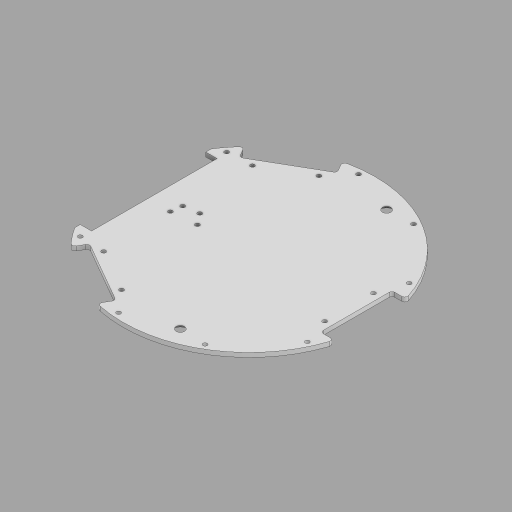
# Autodesk Inventor part: V_1
Saved by Autodesk Inventor 2024.2 (Build 282272000, 272)
## iProperties
Created: 2023-12-06
Part Number: V_1
Material: Типовые
Document SubType Name: Modeling
Designer: Фёдор
Density: 1 g/cm^3
Appearance: По умолчанию
Author: Фёдор
Autodesk Inventor part; units mm, degrees
ref_plane "YZ Plane" through (0, 0, 0) normal (1, 0, 0) x (0, 1, 0)
ref_plane "XZ Plane" through (0, 0, 0) normal (0, 1, 0) x (-1, 0, 0)
ref_plane "XY Plane" through (0, 0, 0) normal (0, 0, 1) x (1, 0, 0)
sketch "Эскиз1" plane through (0, 0, 0) normal (0, 1, 0) x (-1, 0, 0)
  arc A0 (75.6241, 45) -> (63.8377, 60.5702) centre (0, 0) ccw
  line L0 (0, 0) -> (-88, 0) construction
  line L1 (0, 0) -> (44, 76.2102) construction
  line L2 (0, 0) -> (44, -76.2102) construction
  line L3 (75.6241, 45) -> (75.6241, -45)
  arc A1 (75.6241, -45) -> (75.6241, 45) centre (0, 0) ccw construction
  line L4 (15.7099, 77.2104) -> (59.0112, 52.2104)
  line L5 (15.7099, 77.2104) -> (20.2099, 85.0046)
  line L6 (20.2099, 85.0046) -> (63.5112, 60.0046) construction
  line L7 (63.5112, 60.0046) -> (59.0112, 52.2104)
  line L8 (35.7984, 76.0046) -> (37.7984, 79.4687) construction
  line L9 (37.7984, 79.4687) -> (49.9228, 72.4687) construction
  line L10 (49.9228, 72.4687) -> (47.9228, 69.0046) construction
  line L11 (48.1859, 58.4604) -> (14.6859, 0.4367) construction
  line L12 (26.5353, 70.9604) -> (-6.9647, 12.9367) construction
  line L13 (-6.9647, 12.9367) -> (14.6859, 0.4367) construction
  line L14 (20.2099, 85.0046) -> (20.5364, 85.5702)
  line L15 (63.5112, 60.0046) -> (63.8377, 60.5702)
  arc A2 (63.8377, 60.5702) -> (20.5364, 85.5702) centre (0, 0) ccw construction
  arc A3 (20.5364, 85.5702) -> (-84.5368, 24.4444) centre (0, 0) ccw
  arc A4 (63.4379, -60.9888) -> (75.6241, -45) centre (0, 0) ccw
  arc A5 (21.0989, -85.4332) -> (63.4379, -60.9888) centre (0, 0) ccw construction
  arc A6 (-84.5368, 24.4444) -> (-84.5368, -24.4444) centre (0, 0) ccw construction
  arc A7 (-84.5368, -24.4444) -> (21.0989, -85.4332) centre (0, 0) ccw
  line L16 (-83.7211, 25) -> (-74.7211, 25)
  line L17 (-74.7211, -25) -> (-74.7211, 25)
  line L18 (-83.7211, -25) -> (-83.7211, 25) construction
  line L19 (-87.7211, 7) -> (-83.7211, 7) construction
  line L20 (-87.7211, -7) -> (-87.7211, 7) construction
  line L21 (-83.7211, -7) -> (-87.7211, -7) construction
  line L22 (-74.7211, -25) -> (-83.7211, -25)
  line L23 (-83.7211, 25) -> (-84.3742, 25)
  line L24 (-83.7211, -25) -> (-84.3742, -25)
  line L25 (0, 0) -> (-88, 0) construction
  line L26 (-74.7211, 12.5) -> (-7.7211, 12.5) construction
  line L27 (-74.7211, -12.5) -> (-7.7211, -12.5) construction
  line L28 (-7.7211, -12.5) -> (-7.7211, 12.5) construction
  line L29 (20.2099, -85.0046) -> (15.7099, -77.2104)
  line L30 (59.0112, -52.2104) -> (15.7099, -77.2104)
  line L31 (63.5112, -60.0046) -> (20.2099, -85.0046) construction
  line L32 (37.7984, -79.4687) -> (35.7984, -76.0046) construction
  line L33 (49.9228, -72.4687) -> (37.7984, -79.4687) construction
  line L34 (47.9228, -69.0046) -> (49.9228, -72.4687) construction
  line L35 (59.0112, -52.2104) -> (63.5112, -60.0046)
  line L36 (20.2099, -85.0046) -> (20.5364, -85.5702)
  line L37 (63.5112, -60.0046) -> (63.8377, -60.5702)
  line L38 (0, 0) -> (44, -76.2102) construction
  line L39 (26.5353, -70.9604) -> (-6.9647, -12.9367) construction
  line L40 (48.1859, -58.4604) -> (14.6859, -0.4367) construction
  line L41 (14.6859, -0.4367) -> (-6.9647, -12.9367) construction
  line L42 (15.7099, 77.2104) -> (10.7099, 68.5502) construction
  line L43 (10.7099, 68.5502) -> (54.0112, 43.5502) construction
  line L44 (54.0112, 43.5502) -> (59.0112, 52.2104) construction
  line L45 (13.2099, 72.8803) -> (56.5112, 47.8803) construction
  circle A8 centre (49.583, 51.8803) radius 1.5
  circle A9 centre (20.1381, 68.8803) radius 1.5
  circle A10 centre (-69.7211, 17) radius 1.5
  circle A11 centre (-69.7211, -17) radius 1.5
  circle A12 centre (20.1381, -68.8803) radius 1.5
  circle A13 centre (49.583, -51.8803) radius 1.5
  dimension "d0" = 176
  dimension "d1" = 120
  dimension "d2" = 120
  dimension "d9" = 90
  dimension "d14" = 50
  dimension "d15" = 25
  dimension "d16" = 9
  dimension "d18" = 4
  dimension "d19" = 14
  dimension "d20" = 7
  dimension "d21" = 67
  dimension "d22" = 12.5
  dimension "d33" = 360
  dimension "d37" = 10
  dimension "d38" = 3
  dimension "d39" = 8
  dimension "d40" = 3
  dimension "d41" = 8
  dimension "d44" = 360
  dimension "d101" = 75.6241
  constraints: 92 end point, 35 point on circle, 14 centre point, 11 point on line, 10 perpendicular, 2 midpoint, 2 parallel, 2 symmetric about line, 1 coincident, 1 collinear, 1 horizontal, 1 vertical, 101 other
  measures "d0" diameter of A0
  measures "d1" angle of L0 L2
  measures "d2" angle of L0 L1
  measures "d9" distance of L3.start L3.end
  measures "d14" distance of L4.start L4.end
  measures "d15" distance from line of L4.end L1
  measures "d16" distance of L4.start L5.end
  measures "d18" distance between parallel lines of L9 L6
  measures "d19" distance of L8.end L9.end
  measures "d20" distance between parallel lines of L1 L10
  measures "d21" distance of L11.start L11.end
  measures "d22" distance between parallel lines of L11 L1
  measures "d37" distance of L4.start L42.end
  measures "d38" diameter of A8
  measures "d39" distance from line of L44 A8.centre
  measures "d40" diameter of A9
  measures "d41" distance from line of L42 A9.centre
  measures "d101" distance from line of point (0, 0) L3
extrude "Выдавливание1" add sketch "Эскиз1" along normal blind 3
sketch "Эскиз4" plane through (0, 3, 0) normal (0, 1, 0) x (1, 0, 0)
  line L0 (-75.6241, 45) -> (-75.6241, -45) projected
  line L1 (-75.6241, 45) -> (-66.1241, 45)
  line L2 (-66.1241, 45) -> (-66.1241, -45)
  line L3 (-66.1241, -45) -> (-75.6241, -45)
  line L4 (-75.6241, -45) -> (-75.6241, 45)
  point P0 (0, 0)
  dimension "d64" = 9.5
  dimension "d65" = 90
  constraints: 8 end point, 2 parallel, 1 horizontal, 1 perpendicular
  measures "d64" distance of L2.end L3.end
  measures "d65" distance of L1.end L2.end
extrude "Выдавливание3" cut sketch "Эскиз4" against normal through all
fillet "Сопряжение3" radius 2 4 edges at (-63.8377, 1.5, 60.5702) (-20.5364, 1.5, 85.5702) (-59.0112, 1.5, 52.2104) (-15.7099, 1.5, 77.2104)
sketch "Эскиз6" plane through (0, 3, 0) normal (0, 1, 0) x (1, 0, 0)
  circle A0 centre (0, 0) radius 80 construction
  arc A1 (-75.6241, -45) -> (-65.7018, -58.543) centre (0, 0) ccw projected
  line L0 (-62.4765, -58.2124) -> (-60.0112, -53.9425) projected
  line L1 (-57.2792, -53.2104) -> (-17.442, -76.2104) projected
  line L2 (-16.7099, -78.9425) -> (-19.1752, -83.2124) projected
  arc A2 (-17.8488, -86.1709) -> (84.3742, -25) centre (0, 0) ccw projected
  line L3 (84.3742, -25) -> (74.7211, -25) projected
  line L4 (74.7211, -25) -> (74.7211, 25) projected
  line L5 (74.7211, 25) -> (84.3742, 25) projected
  arc A3 (84.3742, 25) -> (-20.5364, 85.5702) centre (0, 0) ccw projected
  line L6 (-20.5364, 85.5702) -> (-15.7099, 77.2104) projected
  line L7 (-15.7099, 77.2104) -> (-59.0112, 52.2104) projected
  line L8 (-59.0112, 52.2104) -> (-63.8377, 60.5702) projected
  arc A4 (-63.8377, 60.5702) -> (-75.6241, 45) centre (0, 0) ccw projected
  line L9 (-75.6241, 45) -> (-66.1241, 45) projected
  line L10 (-66.1241, 45) -> (-66.1241, -45) projected
  line L11 (-66.1241, -45) -> (-75.6241, -45) projected
  circle A5 centre (69.7211, -17) radius 1.5 projected
  circle A6 centre (69.7211, 17) radius 1.5 projected
  circle A7 centre (-49.583, 51.8803) radius 1.5 projected
  circle A8 centre (-20.1381, 68.8803) radius 1.5 projected
  circle A9 centre (-20.1381, -68.8803) radius 1.5 projected
  circle A10 centre (-49.583, -51.8803) radius 1.5 projected
  line L12 (0, 0) -> (44, -76.2102) construction
  circle A11 centre (42, -72.7461) radius 1.5
  line L13 (0, 0) -> (-7.6697, -87.6651) construction
  line L14 (0, 0) -> (79.7551, -37.1904) construction
  circle A12 centre (76.1299, -35.4999) radius 1.5
  line L15 (-7.6697, -87.6651) -> (-7.3211, -83.6804) construction
  circle A13 centre (-7.3211, -83.6804) radius 1.5
  line L16 (74.7211, 0) -> (0, 0) construction
  circle A14 centre (42, 72.7461) radius 1.5
  circle A15 centre (76.1299, 35.4999) radius 1.5
  circle A16 centre (-7.3211, 83.6804) radius 1.5
  circle A17 centre (-66.713, -51.0429) radius 1.5
  arc A18 (-75.6241, -45) -> (-65.7018, -58.543) centre (0, 0) ccw projected
  circle A19 centre (-66.713, 51.0429) radius 1.5
  line L17 (0, 0) -> (0, -144.8354) construction
  arc A20 (-19.1752, -83.2124) -> (-17.8488, -86.1709) centre (-17.4432, -84.2124) ccw projected
  arc A21 (-65.7018, -58.543) -> (-62.4765, -58.2124) centre (-64.2085, -57.2124) ccw projected
  arc A22 (-57.2792, -53.2104) -> (-60.0112, -53.9425) centre (-58.2792, -54.9425) ccw projected
  arc A23 (-16.7099, -78.9425) -> (-17.442, -76.2104) centre (-18.442, -77.9425) ccw projected
  circle A24 centre (0, 0) radius 88 construction
  line L18 (-74.0208, -47.5911) -> (-74.0208, 47.5911) construction
  arc A25 (-72.0208, -45) -> (-73.6957, -48.093) centre (-72.0208, -47) ccw projected
  line L19 (0, 0) -> (-73.6957, -48.093) construction
  arc A26 (-72.0208, -45) -> (-73.6957, -48.093) centre (-72.0208, -47) ccw
  line L20 (-72.0208, -47) -> (-72.0208, -45) construction
  line L21 (0, 0) -> (-69.8898, -53.4735) construction
  point P0 (45.1871, -75.5124)
  dimension "d71" = 8
  dimension "d72" = 120
  dimension "d73" = 60
  dimension "d74" = 3
  dimension "d76" = 25
  dimension "d77" = 25
  dimension "d78" = 3
  dimension "d79" = 4
  dimension "d82" = 4
  dimension "d83" = 3
  dimension "d85" = 3
  dimension "d87" = 3
  dimension "d127" = 5
  dimension "d141" = 95.1823
  dimension "d142" = 123.128
  dimension "d146" = 30
  dimension "d147" = 65
  dimension "d148" = 4
  dimension "d154" = 52.58
  dimension "d155" = 4
  constraints: 20 end point, 11 centre point, 9 point on circle, 5 coincident, 4 point on line, 4 symmetric about line, 4 vertical, 1 concentric, 1 horizontal, 1 midpoint, 1 tangent, 3 other
  measures "d71" radial gap between concentric circles of A0 A2
  measures "d72" angle of L2 L3
  measures "d73" angle of L2 L12
  measures "d74" diameter of A11
  measures "d76" angle of L13 L2
  measures "d77" angle of L3 L14
  measures "d78" diameter of A12
  measures "d79" distance of L14.end A12.centre
  measures "d82" distance of L13.end L15.end
  measures "d83" diameter of A13
  measures "d85" diameter of A17
  measures "d87" diameter of A19
  measures "d127" angle of L13 L17
  measures "d141" distance of L18.start L18.end
  measures "d142" angle of L19 L20
  measures "d146" angle of L12 L17
  measures "d147" angle of L17 L14
  measures "d148" distance of A11.centre L12.end
  measures "d154" angle of L17 L21
  measures "d155" distance of L21.end A17.centre
extrude "Выдавливание4" cut sketch "Эскиз6" against normal through all contours A11 | A12 | A13 | A14 | A15 | A16 | A17 | A19
sketch "Эскиз10" plane through (0, 0, 0) normal (0, -1, 0) x (1, 0, 0)
  circle A0 centre (-50.4241, 4.6) radius 1.5
  circle A1 centre (-49.4241, -3.1) radius 1.5
  circle A2 centre (-33.0241, 3.1) radius 1.5
  circle A3 centre (-39.0241, -4.6) radius 1.5
  line L0 (-27.5241, -8.1) -> (-57.9241, -8.1)
  line L1 (-57.9241, 8.1) -> (-57.9241, -8.1)
  line L2 (-27.5241, 8.1) -> (-57.9241, 8.1)
  line L3 (-27.5241, 8.1) -> (-27.5241, -8.1)
  line L4 (-66.1241, 45) -> (-66.1241, -45) projected
  line L5 (-66.1241, 0) -> (0, 0) construction
  line L6 (-43.9241, 18) -> (-53.9241, 18)
  line L7 (-53.9241, 18) -> (-53.9241, -18)
  line L8 (-53.9241, -18) -> (-43.9241, -18)
  line L9 (-43.9241, -18) -> (-43.9241, 18)
  line L10 (-43.9241, 18) -> (-53.9241, -18) construction
  line L11 (-53.9241, 18) -> (-43.9241, -18) construction
  line L12 (-48.9241, -18) -> (-48.9241, -14) construction
  circle A4 centre (-48.9241, -14) radius 1.5 construction
  circle A5 centre (-48.9241, 14) radius 1.5 construction
  circle A6 centre (0, 0) radius 88
  line L13 (-74.0208, -47.5911) -> (-74.0208, 47.5911)
  arc A7 (-73.6957, 48.093) -> (-72.0208, 45) centre (-72.0208, 47) ccw projected
  arc A8 (-72.0208, -45) -> (-73.6957, -48.093) centre (-72.0208, -47) ccw projected
  point P0 (-66.1241, 43)
  point P1 (-66.1241, -43)
  point P2 (-57.9241, 0)
  point P3 (-48.9241, 0)
  point P4 (-75.6241, -44.4466)
  dimension "d105" = 5
  dimension "d106" = 8.5
  dimension "d107" = 30.4
  dimension "d108" = 16.2
  dimension "d109" = 3.5
  dimension "d110" = 11.5
  dimension "d111" = 5
  dimension "d112" = 5.5
  dimension "d113" = 3.5
  dimension "d114" = 7.5
  dimension "d115" = 8.2
  dimension "d116" = 3
  dimension "d117" = 3
  dimension "d118" = 3
  dimension "d119" = 3
  dimension "d122" = 10
  dimension "d123" = 36
  dimension "d124" = 4
  dimension "d125" = 4
  dimension "d126" = 3
  dimension "d128" = 95.1823
  constraints: 26 end point, 7 centre point, 5 midpoint, 3 perpendicular, 2 coincident, 2 horizontal, 2 parallel, 2 point on circle, 2 point on line, 2 tangent, 2 vertical, 1 symmetric about line, 1 other
  measures "d105" distance from line of L0 A1.centre
  measures "d106" distance from line of L1 A1.centre
  measures "d107" distance between parallel lines of L3 L1
  measures "d108" distance of L2.start L0.start
  measures "d109" distance from line of L0 A3.centre
  measures "d110" distance from line of L3 A3.centre
  measures "d111" distance from line of L2 A2.centre
  measures "d112" distance from line of L3 A2.centre
  measures "d113" distance from line of L2 A0.centre
  measures "d114" distance from line of L1 A0.centre
  measures "d115" distance between parallel lines of L4 L1
  measures "d116" diameter of A1
  measures "d117" diameter of A0
  measures "d118" diameter of A2
  measures "d119" diameter of A3
  measures "d122" distance of L8.end L7.end
  measures "d123" distance of L7.end L6.end
  measures "d124" distance between parallel lines of L1 L7
  measures "d125" distance of L12.start L12.end
  measures "d126" diameter of A4
  measures "d128" distance of L13.start L13.end
extrude "Выдавливание6" cut sketch "Эскиз10" against normal blind 10 contours A0 | A1 | A2 | A3
sketch "Эскиз11" plane through (0, 3, 0) normal (0, 1, 0) x (1, 0, 0)
  arc A0 (-20.5364, -85.5702) -> (84.3742, -25) centre (0, 0) ccw projected
  line L0 (24, -84.664) -> (24, 84.664) construction
  arc A1 (84.3742, 25) -> (-20.5364, 85.5702) centre (0, 0) ccw projected
  circle A2 centre (24, -72) radius 3
  circle A3 centre (24, 72) radius 3
  point P0 (-17.8488, -86.1709)
  point P1 (83.5506, -27.6279)
  point P2 (83.5506, 27.6279)
  point P3 (-17.8488, 86.1709)
  dimension "d129" = 24
  dimension "d130" = 6
  dimension "d131" = 6
  dimension "d132" = 72
  dimension "d133" = 72
  constraints: 2 centre point, 2 end point, 2 point on circle, 2 point on line, 1 vertical
  measures "d129" distance from line of L0 point (0, 0)
  measures "d130" diameter of A2
  measures "d131" diameter of A3
  measures "d132" vertical distance of A2.centre point (0, 0)
  measures "d133" vertical distance of A3.centre point (0, 0)
extrude "Выдавливание7" cut sketch "Эскиз11" against normal blind 10
chamfer "Фаска1" distance 3 angle 45 2 edges at (21, 0, 72) (21, 0, -72)
pattern_circular "Круговой массив3" count 3 over 360 about axis through (0, 0, 0) along (0, 1, 0) of "Сопряжение3"
sketch "Эскиз12" plane through (0, 3, 0) normal (0, 1, 0) x (1, 0, 0)
  arc A0 (-75.6241, -45) -> (-65.7018, -58.543) centre (0, 0) ccw projected
  line L0 (-74.0231, -47.5877) -> (-74.0231, 47.5877)
  arc A1 (-65.7018, 58.543) -> (-75.6241, 45) centre (0, 0) ccw projected
  circle A2 centre (-50.4241, -4.6) radius 1.5 projected
  circle A3 centre (-39.0241, 4.6) radius 1.5 projected
  circle A4 centre (-49.4241, 3.1) radius 1.5 projected
  circle A5 centre (-33.0241, -3.1) radius 1.5 projected
  circle A6 centre (-7.3211, 83.6804) radius 1.5 projected
  circle A7 centre (42, -72.7461) radius 1.5 projected
  circle A8 centre (76.1299, -35.4999) radius 1.5 projected
  circle A9 centre (-66.713, 51.0429) radius 1.5 projected
  circle A10 centre (42, 72.7461) radius 1.5 projected
  circle A11 centre (-7.3211, -83.6804) radius 1.5 projected
  circle A12 centre (76.1299, 35.4999) radius 1.5 projected
  circle A13 centre (-66.713, -51.0429) radius 1.5 projected
  circle A14 centre (-49.583, -51.8803) radius 1.5 projected
  circle A15 centre (-20.1381, -68.8803) radius 1.5 projected
  circle A16 centre (-20.1381, 68.8803) radius 1.5 projected
  circle A17 centre (-49.583, 51.8803) radius 1.5 projected
  circle A18 centre (69.7211, 17) radius 1.5 projected
  circle A19 centre (69.7211, -17) radius 1.5 projected
  arc A20 (-62.4765, 58.2124) -> (-65.7018, 58.543) centre (-64.2085, 57.2124) ccw projected
  arc A21 (-65.7018, 58.543) -> (-75.6241, 45) centre (0, 0) ccw projected
  line L1 (-75.6241, 45) -> (-66.1241, 45) projected
  line L2 (-66.1241, 45) -> (-66.1241, -45) projected
  line L3 (-66.1241, -45) -> (-75.6241, -45) projected
  arc A22 (-75.6241, -45) -> (-65.7018, -58.543) centre (0, 0) ccw projected
  arc A23 (-65.7018, -58.543) -> (-62.4765, -58.2124) centre (-64.2085, -57.2124) ccw projected
  line L4 (-62.4765, -58.2124) -> (-60.0112, -53.9425) projected
  arc A24 (-57.2792, -53.2104) -> (-60.0112, -53.9425) centre (-58.2792, -54.9425) ccw projected
  line L5 (-57.2792, -53.2104) -> (-17.442, -76.2104) projected
  arc A25 (-16.7099, -78.9425) -> (-17.442, -76.2104) centre (-18.442, -77.9425) ccw projected
  line L6 (-16.7099, -78.9425) -> (-19.1752, -83.2124) projected
  arc A26 (-19.1752, -83.2124) -> (-17.8488, -86.1709) centre (-17.4432, -84.2124) ccw projected
  arc A27 (-17.8488, -86.1709) -> (83.5506, -27.6279) centre (0, 0) ccw projected
  arc A28 (83.5506, -27.6279) -> (81.6517, -25) centre (81.6517, -27) ccw projected
  line L7 (81.6517, -25) -> (76.7211, -25) projected
  arc A29 (74.7211, -23) -> (76.7211, -25) centre (76.7211, -23) ccw projected
  line L8 (74.7211, -23) -> (74.7211, 23) projected
  arc A30 (76.7211, 25) -> (74.7211, 23) centre (76.7211, 23) ccw projected
  line L9 (76.7211, 25) -> (81.6517, 25) projected
  arc A31 (81.6517, 25) -> (83.5506, 27.6279) centre (81.6517, 27) ccw projected
  arc A32 (83.5506, 27.6279) -> (-17.8488, 86.1709) centre (0, 0) ccw projected
  arc A33 (-17.8488, 86.1709) -> (-19.1752, 83.2124) centre (-17.4432, 84.2124) ccw projected
  line L10 (-19.1752, 83.2124) -> (-16.7099, 78.9425) projected
  arc A34 (-17.442, 76.2104) -> (-16.7099, 78.9425) centre (-18.442, 77.9425) ccw projected
  line L11 (-17.442, 76.2104) -> (-57.2792, 53.2104) projected
  arc A35 (-60.0112, 53.9425) -> (-57.2792, 53.2104) centre (-58.2792, 54.9425) ccw projected
  line L12 (-60.0112, 53.9425) -> (-62.4765, 58.2124) projected
  point P0 (-74.0231, -45)
  point P1 (-75.6241, 45)
  point P2 (-74.0231, 45)
  dimension "d150" = 1.601
  constraints: 2 end point, 2 point on circle, 1 vertical
  measures "d150" distance from line of A1.end L0
extrude "Выдавливание8" cut sketch "Эскиз12" against normal blind 10 contours L3 L0 A0 | L1 A1 L0
fillet "Сопряжение4" radius 2 2 edges at (-74.0231, 1.5, 47.5877) (-74.0231, 1.5, -47.5877)
sketch "Эскиз13" plane through (0, 3, 0) normal (0, 1, 0) x (1, 0, 0)
  line L0 (-66.1241, -45) -> (-74.0231, -45)
  line L1 (-74.0231, -45) -> (-74.0231, -43.799)
  line L2 (-74.0231, -43.799) -> (-66.1241, -43.799)
  line L3 (-66.1241, -43.799) -> (-66.1241, -45)
  circle A0 centre (69.7211, -17) radius 1.5 projected
  circle A1 centre (69.7211, 17) radius 1.5 projected
  circle A2 centre (-49.583, 51.8803) radius 1.5 projected
  circle A3 centre (-20.1381, 68.8803) radius 1.5 projected
  circle A4 centre (-20.1381, -68.8803) radius 1.5 projected
  circle A5 centre (-49.583, -51.8803) radius 1.5 projected
  circle A6 centre (-66.713, -51.0429) radius 1.5 projected
  circle A7 centre (76.1299, 35.4999) radius 1.5 projected
  circle A8 centre (-7.3211, -83.6804) radius 1.5 projected
  circle A9 centre (42, 72.7461) radius 1.5 projected
  circle A10 centre (-66.713, 51.0429) radius 1.5 projected
  circle A11 centre (76.1299, -35.4999) radius 1.5 projected
  circle A12 centre (42, -72.7461) radius 1.5 projected
  circle A13 centre (-7.3211, 83.6804) radius 1.5 projected
  circle A14 centre (-33.0241, -3.1) radius 1.5 projected
  circle A15 centre (-49.4241, 3.1) radius 1.5 projected
  circle A16 centre (-39.0241, 4.6) radius 1.5 projected
  circle A17 centre (-50.4241, -4.6) radius 1.5 projected
  circle A18 centre (24, 72) radius 3 projected
  circle A19 centre (24, -72) radius 3 projected
  arc A20 (-73.698, 48.0895) -> (-74.0231, 46.9966) centre (-72.0231, 46.9966) ccw projected
  line L4 (-74.0231, 46.9966) -> (-74.0231, 45) projected
  line L5 (-74.0231, 45) -> (-66.1241, 45) projected
  line L6 (-66.1241, 45) -> (-66.1241, -45) projected
  line L7 (-66.1241, -45) -> (-74.0231, -45) projected
  line L8 (-74.0231, -45) -> (-74.0231, -46.9966) projected
  arc A21 (-74.0231, -46.9966) -> (-73.698, -48.0895) centre (-72.0231, -46.9966) ccw projected
  arc A22 (-73.698, -48.0895) -> (-65.7018, -58.543) centre (0, 0) ccw projected
  arc A23 (-65.7018, -58.543) -> (-62.4765, -58.2124) centre (-64.2085, -57.2124) ccw projected
  line L9 (-62.4765, -58.2124) -> (-60.0112, -53.9425) projected
  arc A24 (-57.2792, -53.2104) -> (-60.0112, -53.9425) centre (-58.2792, -54.9425) ccw projected
  line L10 (-57.2792, -53.2104) -> (-17.442, -76.2104) projected
  arc A25 (-16.7099, -78.9425) -> (-17.442, -76.2104) centre (-18.442, -77.9425) ccw projected
  line L11 (-16.7099, -78.9425) -> (-19.1752, -83.2124) projected
  arc A26 (-19.1752, -83.2124) -> (-17.8488, -86.1709) centre (-17.4432, -84.2124) ccw projected
  arc A27 (-17.8488, -86.1709) -> (83.5506, -27.6279) centre (0, 0) ccw projected
  arc A28 (83.5506, -27.6279) -> (81.6517, -25) centre (81.6517, -27) ccw projected
  line L12 (81.6517, -25) -> (76.7211, -25) projected
  arc A29 (74.7211, -23) -> (76.7211, -25) centre (76.7211, -23) ccw projected
  line L13 (74.7211, -23) -> (74.7211, 23) projected
  arc A30 (76.7211, 25) -> (74.7211, 23) centre (76.7211, 23) ccw projected
  line L14 (76.7211, 25) -> (81.6517, 25) projected
  arc A31 (81.6517, 25) -> (83.5506, 27.6279) centre (81.6517, 27) ccw projected
  arc A32 (83.5506, 27.6279) -> (-17.8488, 86.1709) centre (0, 0) ccw projected
  arc A33 (-17.8488, 86.1709) -> (-19.1752, 83.2124) centre (-17.4432, 84.2124) ccw projected
  line L15 (-19.1752, 83.2124) -> (-16.7099, 78.9425) projected
  arc A34 (-17.442, 76.2104) -> (-16.7099, 78.9425) centre (-18.442, 77.9425) ccw projected
  line L16 (-17.442, 76.2104) -> (-57.2792, 53.2104) projected
  arc A35 (-60.0112, 53.9425) -> (-57.2792, 53.2104) centre (-58.2792, 54.9425) ccw projected
  line L17 (-60.0112, 53.9425) -> (-62.4765, 58.2124) projected
  arc A36 (-62.4765, 58.2124) -> (-65.7018, 58.543) centre (-64.2085, 57.2124) ccw projected
  arc A37 (-65.7018, 58.543) -> (-73.698, 48.0895) centre (0, 0) ccw projected
  line L18 (-74.0231, -45) -> (-74.0231, -46.9966) projected
  line L19 (-66.1241, 0) -> (74.7211, 0) construction
  line L20 (-66.1241, 45) -> (-74.0231, 45)
  line L21 (-74.0231, 45) -> (-74.0231, 43.799)
  line L22 (-74.0231, 43.799) -> (-66.1241, 43.799)
  line L23 (-66.1241, 43.799) -> (-66.1241, 45)
  line L24 (-66.1241, 45) -> (-74.0231, 45)
  line L25 (-74.0231, 45) -> (-74.0231, 46.9966)
  line L26 (-74.0231, 45) -> (-74.0231, 46.9966)
  point P0 (-70.0736, -43.799)
  point P1 (-72.0231, 46.9966)
  point P2 (-70.0736, 43.799)
  dimension "d156" = 1.201
  constraints: 24 end point, 8 symmetric about line, 3 midpoint, 2 parallel, 1 collinear, 1 horizontal, 1 perpendicular
  measures "d156" distance from line of point (-70.074, -43.799) L0
extrude "Выдавливание9" add sketch "Эскиз13" against normal blind 3 contours L0 L1 L2 L3 | L22 L21 L5 L6
equation "\"d15\" = 0.5 * d14"
equation "\"d133\" = d132"
